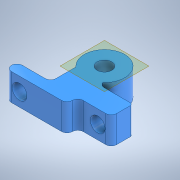
# Autodesk Inventor part: 4mm_Roller_Spacer
Saved by Autodesk Inventor 2021 (Build 250183000, 183)
## iProperties
Created: 2021-03-29
Part Number: 4mm_Roller_Spacer
Material: PET Plastic
Document SubType Name: Modeling
Designer: Jorian Brusind
Density: 1.541 g/cm^3
Appearance: Cyan
Author: Jorian Brusind
Autodesk Inventor part; units mm, degrees
ref_plane "YZ Plane" through (0, 0, 0) normal (1, 0, 0) x (0, 1, 0)
ref_plane "XZ Plane" through (0, 0, 0) normal (0, 1, 0) x (-1, 0, 0)
ref_plane "XY Plane" through (0, 0, 0) normal (0, 0, 1) x (1, 0, 0)
sketch "Sketch4" plane through (0, 0, 0) normal (0, 1, 0) x (-1, 0, 0)
  circle A0 centre (0, 0) radius 7.5
  circle A1 centre (0, 0) radius 2.75
  dimension "d19" = 15
  dimension "d20" = 5.5
  constraints: 2 centre point, 2 coincident
  measures "d19" diameter of A0
  measures "d20" diameter of A1
extrude "Extrusion4" add sketch "Sketch4" along normal blind 10
ref_plane "Work Plane1" through (0, 10, 0) normal (0, -1, 0) x (1, 0, 0)
sketch "Sketch7" plane through (0, 10, 0) normal (0, -1, 0) x (1, 0, 0)
  line L0 (0, 0) -> (0, 15)
  line L1 (17.5, 19) -> (-17.5, 19)
  line L2 (-17.5, 19) -> (-17.5, 11)
  line L3 (-17.5, 11) -> (17.5, 11)
  line L4 (17.5, 11) -> (17.5, 19)
  line L5 (17.5, 19) -> (-17.5, 11) construction
  line L6 (-17.5, 19) -> (17.5, 11) construction
  line L7 (5, 24.41) -> (-5, 24.41)
  line L8 (-5, 24.41) -> (-5, 5.59)
  line L9 (-5, 5.59) -> (5, 5.59)
  line L10 (5, 5.59) -> (5, 24.41)
  line L11 (5, 24.41) -> (-5, 5.59) construction
  line L12 (-5, 24.41) -> (5, 5.59) construction
  point P0 (-5, 11)
  point P1 (5, 11)
  dimension "d35" = 15
  dimension "d36" = 35
  dimension "d37" = 8
  dimension "d38" = 10
  dimension "d39" = 18.82
  constraints: 26 end point, 4 midpoint, 4 parallel, 2 horizontal, 2 perpendicular, 1 vertical
  measures "d35" distance of L0.start L0.end
  measures "d36" distance of L3.end L2.end
  measures "d37" distance of L2.end L1.end
  measures "d38" distance of L9.end L8.end
  measures "d39" distance of L8.end L7.end
extrude "Extrusion6" add sketch "Sketch7" along normal up to surface (10 mm away) contours L9 L8 L3 L0 | L0 L3 L10 L9 | L3 L8 L1 L10 | L3 L2 L1 L8 | L10 L1 L4 L3
sketch "Sketch8" plane through (-5, 10, 11) normal (0, 0, -1) x (-1, 0, 0)
  point P0 (-5, -10)
move faces "Move2" translate (0, 0, 4) faces at (-13.3333, 6.6667, 11) (1.6667, 0, 16.3333)
sketch "Sketch9" plane through (-17.5, 10, 19) normal (0, 0, 1) x (1, 0, 0)
  line L0 (35, 0) -> (35, -10) projected
  line L1 (35, -10) -> (0, -10) projected
  line L2 (35, 0) -> (22.5799, 0)
  line L3 (22.5799, 0) -> (22.5799, -10)
  line L4 (22.5799, -10) -> (35, -10)
  line L5 (35, -10) -> (35, 0)
  point P0 (17.5, -10)
  constraints: 8 end point, 2 parallel, 1 horizontal, 1 perpendicular, 1 point on line
extrude "Extrusion7" cut sketch "Sketch9" against normal blind 4
sketch "Sketch10" plane through (17.5, 10, 11) normal (0, 0, -1) x (-1, 0, 0)
  circle A0 centre (5, -5) radius 2.75
  circle A1 centre (30, -5) radius 2.75
  line L0 (35, -10) -> (22.5, -10) projected
  line L1 (35, 0) -> (35, -10) projected
  line L2 (0, 0) -> (0, -10) projected
  line L3 (12.5, -10) -> (0, -10) projected
  point P0 (17.5, -10)
  dimension "d50" = 5.5
  dimension "d51" = 5.5
  dimension "d52" = 5
  dimension "d53" = 5
  dimension "d54" = 5
  dimension "d55" = 5
  constraints: 2 centre point
  measures "d50" diameter of A0
  measures "d51" diameter of A1
  measures "d52" distance from line of L0 A1.centre
  measures "d53" distance from line of L1 A1.centre
  measures "d54" distance from line of L2 A0.centre
  measures "d55" distance from line of L3 A0.centre
extrude "Extrusion8" cut sketch "Sketch10" against normal through all
sketch "Sketch11" plane through (17.5, 10, 11) normal (0, 0, -1) x (-1, 0, 0)
  circle A0 centre (5, -5) radius 2.75 projected
  line L0 (5, -9.6188) -> (1, -7.3094)
  line L1 (1, -7.3094) -> (1, -2.6906)
  line L2 (1, -2.6906) -> (5, -0.3812)
  line L3 (5, -0.3812) -> (9, -2.6906)
  line L4 (9, -2.6906) -> (9, -7.3094)
  line L5 (9, -7.3094) -> (5, -9.6188)
  line L6 (0, 0) -> (0, -10) projected
  line L7 (12.5, 0) -> (12.5, -10) projected
  line L8 (0, 0) -> (12.5, 0)
  line L9 (12.5, 0) -> (12.5, -10)
  line L10 (12.5, -10) -> (0, -10)
  line L11 (0, -10) -> (0, 0)
  point P0 (17.5, -10)
  point P1 (12.4201, 0)
  dimension "d58" = 8
  constraints: 20 end point, 2 parallel, 1 coincident, 1 horizontal, 1 perpendicular, 13 other
  measures "d58" distance between parallel lines of L1 L4
extrude "Extrusion9" add sketch "Sketch11" along normal blind 4 contours L8 L7 L10 L6
fillet "Fillet1" radius 2 5 edges at (-17.5, 5, 15) (17.5, 5, 15) (5.0799, 5, 19) (5.0799, 5, 15) (-17.5, 5, 19)
fillet "Fillet2" radius 1 1 edges at (17.5, 5, 7)
fillet "Fillet3" radius 2 2 edges at (5, 5, 7) (-5, 5, 15)
body "Solid2"
